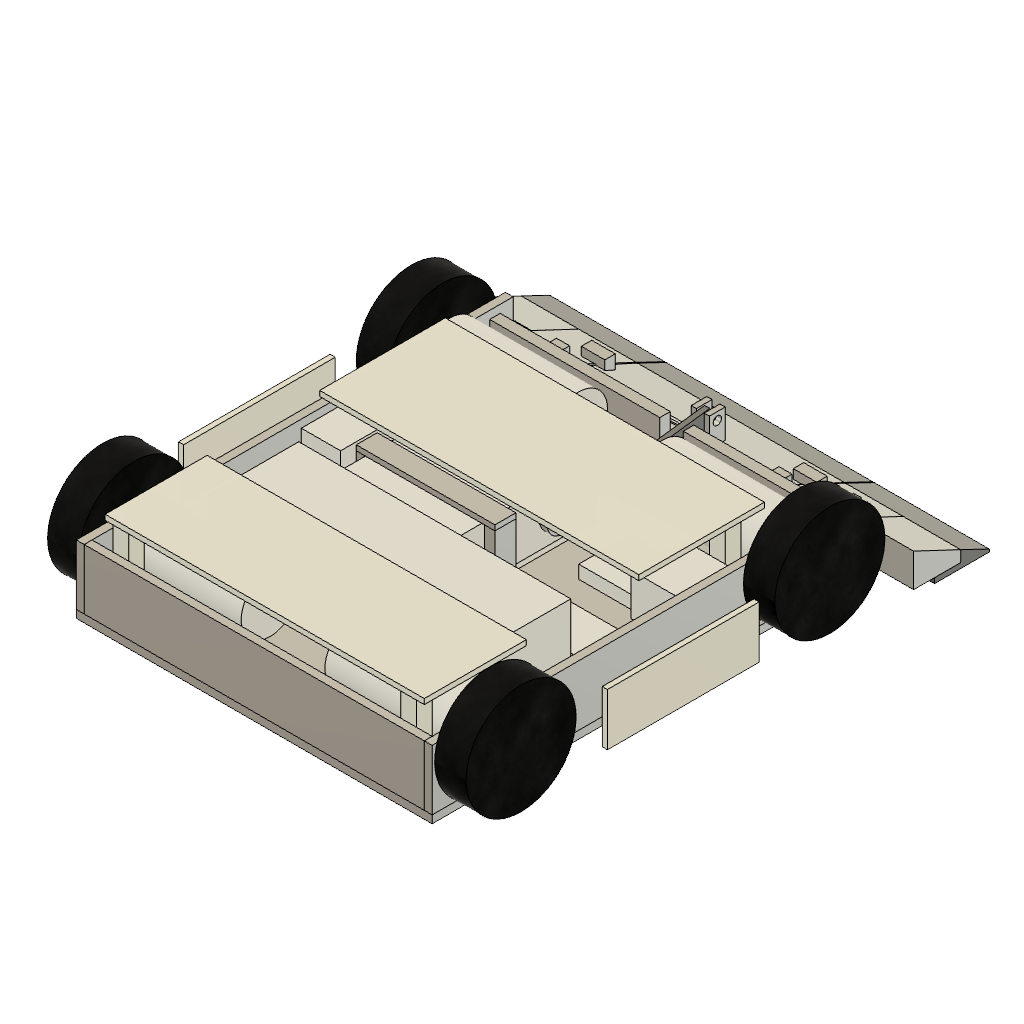
ROBOT_V3_R3_Lifter (Autodesk Fusion 360 design; units mm, degrees)
part number: 2026-09-25-01-00-55-183
part number: 2026-09-25-01-00-55-288
part number: 2026-09-25-01-00-55-293
part number: 2026-09-25-01-00-55-304
part number: 2026-09-25-01-00-55-313
part number: 2026-09-25-01-00-55-323
part number: 2026-09-25-01-00-55-333
part number: 2026-09-25-01-00-55-343
part number: 2026-09-25-01-00-55-353
part number: 2026-09-25-01-00-55-375
part number: 2026-09-25-01-00-55-378
part number: 2026-09-25-01-00-55-389
part number: 2026-09-25-01-00-55-400
part number: 2026-09-25-01-00-55-412
part number: 2026-09-25-01-00-55-424
part number: 2026-09-25-01-00-55-437
part number: 2026-09-25-01-00-55-451
part number: 2026-09-25-01-00-55-467
part number: 2026-09-25-01-00-55-483
part number: 2026-09-25-01-00-55-502
part number: 2026-09-25-01-00-55-522
part number: 2026-09-25-01-00-55-527
part number: 2026-09-25-01-00-55-700
part number: 2026-09-25-01-00-55-756
part number: 2026-09-25-01-00-55-814
part number: 2026-09-25-01-00-55-881
part number: 2026-09-25-01-00-55-947
part number: 2026-09-25-01-00-56-020
part number: 2026-09-25-01-00-56-029
part number: 2026-09-25-01-00-56-371
part number: 2026-09-25-01-00-56-429
part number: 2026-09-25-01-00-56-469
part number: 2026-09-25-01-00-56-511
part number: 2026-09-25-01-00-56-554
part number: 2026-09-25-01-00-56-599
part number: 2026-09-25-01-00-56-645
part number: 2026-09-25-01-00-56-689
part number: 2026-09-25-01-00-56-777
part number: 2026-09-25-01-00-56-983
part number: 2026-09-25-01-00-56-997
part number: 2026-09-25-01-00-57-050
part number: 2026-09-25-01-00-57-102
part number: 2026-09-25-01-00-57-155
part number: 2026-09-25-01-00-57-208
part number: 2026-09-25-01-00-57-261
part number: 2026-09-25-01-00-57-276
part number: 2026-09-25-01-00-57-328
part number: 2026-09-25-01-00-57-386
part number: 2026-09-25-01-00-57-443
part number: 2026-09-25-01-00-57-501
part number: 2026-09-25-01-00-57-558
Autodesk Fusion 360 part; units mm, degrees
sketch "Base_6061_3mm_Footprint" plane through (0, 0, 0) normal (0, 1, 0) x (1, 0, 0) in component "Base_6061_3mm"
  line L0 (-68, -82) -> (68, -82)
  line L1 (68, -82) -> (68, 74)
  line L2 (68, 74) -> (-68, 74)
  line L3 (-68, 74) -> (-68, -82)
extrude "Extrude1" add sketch "Base_6061_3mm_Footprint" along normal blind 3 from surface at 3 makes body 1 in component "Base_6061_3mm"
sketch "Base_Wing_Tab_L_Footprint" plane through (0, 0, 0) normal (0, 1, 0) x (1, 0, 0) in component "Base_Wing_Tab_L"
  line L0 (-68, 74) -> (-41, 74)
  line L1 (-41, 74) -> (-41, 82)
  line L2 (-41, 82) -> (-68, 82)
  line L3 (-68, 82) -> (-68, 74)
extrude "Extrude1'" add sketch "Base_Wing_Tab_L_Footprint" along normal blind 3 from surface at 3 separate body makes body 2 in component "Base_Wing_Tab_L"
sketch "Base_Wing_Tab_R_Footprint" plane through (0, 0, 0) normal (0, 1, 0) x (1, 0, 0) in component "Base_Wing_Tab_R"
  line L0 (41, 74) -> (68, 74)
  line L1 (68, 74) -> (68, 82)
  line L2 (68, 82) -> (41, 82)
  line L3 (41, 82) -> (41, 74)
extrude "Extrude1''" add sketch "Base_Wing_Tab_R_Footprint" along normal blind 3 from surface at 3 separate body makes body 3 in component "Base_Wing_Tab_R"
sketch "Side_Rail_L_6061_Footprint" plane through (0, 0, 0) normal (0, 1, 0) x (1, 0, 0) in component "Side_Rail_L_6061"
  line L0 (-68, -82) -> (-65, -82)
  line L1 (-65, -82) -> (-65, 82)
  line L2 (-65, 82) -> (-68, 82)
  line L3 (-68, 82) -> (-68, -82)
extrude "Extrude1'''" add sketch "Side_Rail_L_6061_Footprint" along normal blind 23 from surface at 6 separate body makes body 4 in component "Side_Rail_L_6061"
sketch "Side_Rail_R_6061_Footprint" plane through (0, 0, 0) normal (0, 1, 0) x (1, 0, 0) in component "Side_Rail_R_6061"
  line L0 (65, -82) -> (68, -82)
  line L1 (68, -82) -> (68, 82)
  line L2 (68, 82) -> (65, 82)
  line L3 (65, 82) -> (65, -82)
extrude "Extrude1''''" add sketch "Side_Rail_R_6061_Footprint" along normal blind 23 from surface at 6 separate body makes body 5 in component "Side_Rail_R_6061"
sketch "Rear_Cross_Member_6061_Footprint" plane through (0, 0, 0) normal (0, 1, 0) x (1, 0, 0) in component "Rear_Cross_Member_6061"
  line L0 (-65, -82) -> (65, -82)
  line L1 (65, -82) -> (65, -79)
  line L2 (65, -79) -> (-65, -79)
  line L3 (-65, -79) -> (-65, -82)
extrude "Extrude1'''''" add sketch "Rear_Cross_Member_6061_Footprint" along normal blind 23 from surface at 6 separate body makes body 6 in component "Rear_Cross_Member_6061"
sketch "Front_Impact_Bulkhead_6061_Footprint" plane through (0, 0, 0) normal (0, 1, 0) x (1, 0, 0) in component "Front_Impact_Bulkhead_6061"
  line L0 (-62, 70) -> (62, 70)
  line L1 (62, 70) -> (62, 74)
  line L2 (62, 74) -> (-62, 74)
  line L3 (-62, 74) -> (-62, 70)
extrude "Extrude1''''''" add sketch "Front_Impact_Bulkhead_6061_Footprint" along normal blind 23 from surface at 6 separate body makes body 7 in component "Front_Impact_Bulkhead_6061"
sketch "Pushrod_Slot" plane through (0, 0, 0) normal (1, 0, 0) x (0, 0, -1) in component "Front_Impact_Bulkhead_6061"
  line L0 (69, 14) -> (69, 30)
  line L1 (69, 30) -> (75, 30)
  line L2 (75, 30) -> (75, 14)
  line L3 (75, 14) -> (69, 14)
extrude "Extrude2" cut sketch "Pushrod_Slot" along normal blind 9 from surface at 3 bodies 7 in component "Front_Impact_Bulkhead_6061"
sketch "BBB_22mm_Gearmotor_ENVELOPE_L_Rear_Section" plane through (0, 0, 0) normal (1, 0, 0) x (0, 0, -1) in component "BBB_22mm_Gearmotor_ENVELOPE_L_Rear"
  circle A0 centre (-60, 23) radius 11
extrude "Extrude1'''''''" add sketch "BBB_22mm_Gearmotor_ENVELOPE_L_Rear_Section" along normal blind 49 from surface at -65 separate body makes body 8 in component "BBB_22mm_Gearmotor_ENVELOPE_L_Rear"
sketch "Wheel_42mm_ENVELOPE_L_Rear_Section" plane through (0, 0, 0) normal (1, 0, 0) x (0, 0, -1) in component "Wheel_42mm_ENVELOPE_L_Rear"
  circle A0 centre (-60, 23) radius 21
extrude "Extrude1''''''''" add sketch "Wheel_42mm_ENVELOPE_L_Rear_Section" along normal blind 12 from surface at -80 separate body makes body 9 in component "Wheel_42mm_ENVELOPE_L_Rear"
sketch "BBB_22mm_Gearmotor_ENVELOPE_L_Front_Section" plane through (0, 0, 0) normal (1, 0, 0) x (0, 0, -1) in component "BBB_22mm_Gearmotor_ENVELOPE_L_Front"
  circle A0 centre (58, 23) radius 11
extrude "Extrude1'''''''''" add sketch "BBB_22mm_Gearmotor_ENVELOPE_L_Front_Section" along normal blind 49 from surface at -65 separate body makes body 10 in component "BBB_22mm_Gearmotor_ENVELOPE_L_Front"
sketch "Wheel_42mm_ENVELOPE_L_Front_Section" plane through (0, 0, 0) normal (1, 0, 0) x (0, 0, -1) in component "Wheel_42mm_ENVELOPE_L_Front"
  circle A0 centre (58, 23) radius 21
extrude "Extrude1''''''''''" add sketch "Wheel_42mm_ENVELOPE_L_Front_Section" along normal blind 12 from surface at -80 separate body makes body 11 in component "Wheel_42mm_ENVELOPE_L_Front"
sketch "BBB_22mm_Gearmotor_ENVELOPE_R_Rear_Section" plane through (0, 0, 0) normal (1, 0, 0) x (0, 0, -1) in component "BBB_22mm_Gearmotor_ENVELOPE_R_Rear"
  circle A0 centre (-60, 23) radius 11
extrude "Extrude1'''''''''''" add sketch "BBB_22mm_Gearmotor_ENVELOPE_R_Rear_Section" along normal blind 49 from surface at 16 separate body makes body 12 in component "BBB_22mm_Gearmotor_ENVELOPE_R_Rear"
sketch "Wheel_42mm_ENVELOPE_R_Rear_Section" plane through (0, 0, 0) normal (1, 0, 0) x (0, 0, -1) in component "Wheel_42mm_ENVELOPE_R_Rear"
  circle A0 centre (-60, 23) radius 21
extrude "Extrude1''''''''''''" add sketch "Wheel_42mm_ENVELOPE_R_Rear_Section" along normal blind 12 from surface at 68 separate body makes body 13 in component "Wheel_42mm_ENVELOPE_R_Rear"
sketch "BBB_22mm_Gearmotor_ENVELOPE_R_Front_Section" plane through (0, 0, 0) normal (1, 0, 0) x (0, 0, -1) in component "BBB_22mm_Gearmotor_ENVELOPE_R_Front"
  circle A0 centre (58, 23) radius 11
extrude "Extrude1'''''''''''''" add sketch "BBB_22mm_Gearmotor_ENVELOPE_R_Front_Section" along normal blind 49 from surface at 16 separate body makes body 14 in component "BBB_22mm_Gearmotor_ENVELOPE_R_Front"
sketch "Wheel_42mm_ENVELOPE_R_Front_Section" plane through (0, 0, 0) normal (1, 0, 0) x (0, 0, -1) in component "Wheel_42mm_ENVELOPE_R_Front"
  circle A0 centre (58, 23) radius 21
extrude "Extrude1''''''''''''''" add sketch "Wheel_42mm_ENVELOPE_R_Front_Section" along normal blind 12 from surface at 68 separate body makes body 15 in component "Wheel_42mm_ENVELOPE_R_Front"
sketch "Replaceable_Side_Guard_L_Footprint" plane through (0, 0, 0) normal (0, 1, 0) x (1, 0, 0) in component "Replaceable_Side_Guard_L"
  line L0 (-82, -29) -> (-80, -29)
  line L1 (-80, -29) -> (-80, 29)
  line L2 (-80, 29) -> (-82, 29)
  line L3 (-82, 29) -> (-82, -29)
extrude "Extrude1'''''''''''''''" add sketch "Replaceable_Side_Guard_L_Footprint" along normal blind 20 from surface at 8 separate body makes body 16 in component "Replaceable_Side_Guard_L"
sketch "Replaceable_Side_Guard_R_Footprint" plane through (0, 0, 0) normal (0, 1, 0) x (1, 0, 0) in component "Replaceable_Side_Guard_R"
  line L0 (80, -29) -> (82, -29)
  line L1 (82, -29) -> (82, 29)
  line L2 (82, 29) -> (80, 29)
  line L3 (80, 29) -> (80, -29)
extrude "Extrude1''''''''''''''''" add sketch "Replaceable_Side_Guard_R_Footprint" along normal blind 20 from surface at 8 separate body makes body 17 in component "Replaceable_Side_Guard_R"
sketch "Wing_Root_Profile" plane through (0, 0, 0) normal (1, 0, 0) x (0, 0, -1) in component "Fixed_Plow_Wings_6061"
  line L0 (74, 6) -> (74, 23)
  line L1 (74, 23) -> (104, 8.79)
  line L2 (104, 8.79) -> (104, 4.5)
  line L3 (104, 4.5) -> (94, 4.5)
  line L4 (94, 4.5) -> (82, 6)
  line L5 (82, 6) -> (74, 6)
extrude "Extrude1'''''''''''''''''" add sketch "Wing_Root_Profile" along normal blind 22 from surface at -62 separate body makes body 18 in component "Fixed_Plow_Wings_6061"
sketch "Wing_Outer_Profile" plane through (0, 0, 0) normal (1, 0, 0) x (0, 0, -1) in component "Fixed_Plow_Wings_6061"
  line L0 (86, 4.5) -> (86, 17.3)
  line L1 (86, 17.3) -> (104, 8.79)
  line L2 (104, 8.79) -> (104, 4.5)
  line L3 (104, 4.5) -> (86, 4.5)
extrude "Extrude2'" add sketch "Wing_Outer_Profile" along normal blind 22 from surface at -84 bodies 18 in component "Fixed_Plow_Wings_6061"
sketch "Up_Stop_Block" plane through (0, 0, 0) normal (1, 0, 0) x (0, 0, -1) in component "Fixed_Plow_Wings_6061"
  line L0 (74, 23) -> (74, 27)
  line L1 (74, 27) -> (78.54, 27)
  line L2 (78.54, 27) -> (78.54, 20.8496)
  line L3 (78.54, 20.8496) -> (74, 23)
extrude "Extrude3" add sketch "Up_Stop_Block" along normal blind 5 from surface at -45 bodies 18 in component "Fixed_Plow_Wings_6061"
sketch "Pivot_Bore_6p4mm" plane through (0, 0, 0) normal (1, 0, 0) x (0, 0, -1) in component "Fixed_Plow_Wings_6061"
  circle A0 centre (80.5, 13) radius 3.2
extrude "Extrude4" cut sketch "Pivot_Bore_6p4mm" along normal blind 6.5 from surface at -46.5 bodies 18 in component "Fixed_Plow_Wings_6061"
sketch "Wing_Root_Profile (1)" plane through (0, 0, 0) normal (1, 0, 0) x (0, 0, -1) in component "Fixed_Plow_Wings_6061"
  line L0 (74, 6) -> (74, 23)
  line L1 (74, 23) -> (104, 8.79)
  line L2 (104, 8.79) -> (104, 4.5)
  line L3 (104, 4.5) -> (94, 4.5)
  line L4 (94, 4.5) -> (82, 6)
  line L5 (82, 6) -> (74, 6)
extrude "Extrude5" add sketch "Wing_Root_Profile (1)" along normal blind 22 from surface at 40 separate body makes body 19 in component "Fixed_Plow_Wings_6061"
sketch "Wing_Outer_Profile (1)" plane through (0, 0, 0) normal (1, 0, 0) x (0, 0, -1) in component "Fixed_Plow_Wings_6061"
  line L0 (86, 4.5) -> (86, 17.3)
  line L1 (86, 17.3) -> (104, 8.79)
  line L2 (104, 8.79) -> (104, 4.5)
  line L3 (104, 4.5) -> (86, 4.5)
extrude "Extrude6" add sketch "Wing_Outer_Profile (1)" along normal blind 22 from surface at 62 bodies 19 in component "Fixed_Plow_Wings_6061"
sketch "Up_Stop_Block (1)" plane through (0, 0, 0) normal (1, 0, 0) x (0, 0, -1) in component "Fixed_Plow_Wings_6061"
  line L0 (74, 23) -> (74, 27)
  line L1 (74, 27) -> (78.54, 27)
  line L2 (78.54, 27) -> (78.54, 20.8496)
  line L3 (78.54, 20.8496) -> (74, 23)
extrude "Extrude7" add sketch "Up_Stop_Block (1)" along normal blind 5 from surface at 40 bodies 19 in component "Fixed_Plow_Wings_6061"
sketch "Pivot_Bore_6p4mm (1)" plane through (0, 0, 0) normal (1, 0, 0) x (0, 0, -1) in component "Fixed_Plow_Wings_6061"
  circle A0 centre (80.5, 13) radius 3.2
extrude "Extrude8" cut sketch "Pivot_Bore_6p4mm (1)" along normal blind 6.5 from surface at 39.5 bodies 19 in component "Fixed_Plow_Wings_6061"
sketch "Wing_Edge_Profile" plane through (0, 0, 0) normal (1, 0, 0) x (0, 0, -1) in component "Wing_Steel_Edges"
  line L0 (94, 2.5) -> (94, 4.5)
  line L1 (94, 4.5) -> (104, 4.5)
  line L2 (104, 4.5) -> (104, 8.79)
  line L3 (104, 8.79) -> (115, 3.5)
  line L4 (115, 3.5) -> (115, 2.5)
  line L5 (115, 2.5) -> (94, 2.5)
extrude "Extrude1''''''''''''''''''" add sketch "Wing_Edge_Profile" along normal blind 44 from surface at -84 separate body makes body 20 in component "Wing_Steel_Edges"
sketch "Wing_Edge_Profile (1)" plane through (0, 0, 0) normal (1, 0, 0) x (0, 0, -1) in component "Wing_Steel_Edges"
  line L0 (94, 2.5) -> (94, 4.5)
  line L1 (94, 4.5) -> (104, 4.5)
  line L2 (104, 4.5) -> (104, 8.79)
  line L3 (104, 8.79) -> (115, 3.5)
  line L4 (115, 3.5) -> (115, 2.5)
  line L5 (115, 2.5) -> (94, 2.5)
extrude "Extrude2''" add sketch "Wing_Edge_Profile (1)" along normal blind 44 from surface at 40 separate body makes body 21 in component "Wing_Steel_Edges"
sketch "M3x20_Bolt_ENVELOPE_x-49.5_Section" plane through (0, 0, 0) normal (0, 0, 1) x (1, 0, 0) in component "M3x20_Bolt_ENVELOPE_x-49.5"
  circle A0 centre (-49.5, 10) radius 1.5
extrude "Extrude1'''''''''''''''''''" add sketch "M3x20_Bolt_ENVELOPE_x-49.5_Section" along normal blind 19 from surface at -86 separate body makes body 22 in component "M3x20_Bolt_ENVELOPE_x-49.5"
sketch "Bolt_Clearance_x-49.5" plane through (0, 0, 0) normal (0, 0, 1) x (1, 0, 0) in component "Front_Impact_Bulkhead_6061"
  circle A0 centre (-49.5, 10) radius 1.7
extrude "Extrude3'" cut sketch "Bolt_Clearance_x-49.5" along normal blind 5 from surface at -74.5 bodies 7 in component "Front_Impact_Bulkhead_6061"
sketch "Bolt_Tapped_x-49.5" plane through (0, 0, 0) normal (0, 0, 1) x (1, 0, 0) in component "Fixed_Plow_Wings_6061"
  circle A0 centre (-49.5, 10) radius 1.5
extrude "Extrude9" cut sketch "Bolt_Tapped_x-49.5" along normal blind 12 from surface at -86 bodies 18 in component "Fixed_Plow_Wings_6061"
sketch "M3x20_Bolt_ENVELOPE_x-58.5_Section" plane through (0, 0, 0) normal (0, 0, 1) x (1, 0, 0) in component "M3x20_Bolt_ENVELOPE_x-58.5"
  circle A0 centre (-58.5, 10) radius 1.5
extrude "Extrude1''''''''''''''''''''" add sketch "M3x20_Bolt_ENVELOPE_x-58.5_Section" along normal blind 19 from surface at -86 separate body makes body 23 in component "M3x20_Bolt_ENVELOPE_x-58.5"
sketch "Bolt_Clearance_x-58.5" plane through (0, 0, 0) normal (0, 0, 1) x (1, 0, 0) in component "Front_Impact_Bulkhead_6061"
  circle A0 centre (-58.5, 10) radius 1.7
extrude "Extrude4'" cut sketch "Bolt_Clearance_x-58.5" along normal blind 5 from surface at -74.5 bodies 7 in component "Front_Impact_Bulkhead_6061"
sketch "Bolt_Tapped_x-58.5" plane through (0, 0, 0) normal (0, 0, 1) x (1, 0, 0) in component "Fixed_Plow_Wings_6061"
  circle A0 centre (-58.5, 10) radius 1.5
extrude "Extrude10" cut sketch "Bolt_Tapped_x-58.5" along normal blind 12 from surface at -86 bodies 18 in component "Fixed_Plow_Wings_6061"
sketch "M3x20_Bolt_ENVELOPE_x+49.5_Section" plane through (0, 0, 0) normal (0, 0, 1) x (1, 0, 0) in component "M3x20_Bolt_ENVELOPE_x+49.5"
  circle A0 centre (49.5, 10) radius 1.5
extrude "Extrude1'''''''''''''''''''''" add sketch "M3x20_Bolt_ENVELOPE_x+49.5_Section" along normal blind 19 from surface at -86 separate body makes body 24 in component "M3x20_Bolt_ENVELOPE_x+49.5"
sketch "Bolt_Clearance_x+49.5" plane through (0, 0, 0) normal (0, 0, 1) x (1, 0, 0) in component "Front_Impact_Bulkhead_6061"
  circle A0 centre (49.5, 10) radius 1.7
extrude "Extrude5'" cut sketch "Bolt_Clearance_x+49.5" along normal blind 5 from surface at -74.5 bodies 7 in component "Front_Impact_Bulkhead_6061"
sketch "Bolt_Tapped_x+49.5" plane through (0, 0, 0) normal (0, 0, 1) x (1, 0, 0) in component "Fixed_Plow_Wings_6061"
  circle A0 centre (49.5, 10) radius 1.5
extrude "Extrude11" cut sketch "Bolt_Tapped_x+49.5" along normal blind 12 from surface at -86 bodies 19 in component "Fixed_Plow_Wings_6061"
sketch "M3x20_Bolt_ENVELOPE_x+58.5_Section" plane through (0, 0, 0) normal (0, 0, 1) x (1, 0, 0) in component "M3x20_Bolt_ENVELOPE_x+58.5"
  circle A0 centre (58.5, 10) radius 1.5
extrude "Extrude1''''''''''''''''''''''" add sketch "M3x20_Bolt_ENVELOPE_x+58.5_Section" along normal blind 19 from surface at -86 separate body makes body 25 in component "M3x20_Bolt_ENVELOPE_x+58.5"
sketch "Bolt_Clearance_x+58.5" plane through (0, 0, 0) normal (0, 0, 1) x (1, 0, 0) in component "Front_Impact_Bulkhead_6061"
  circle A0 centre (58.5, 10) radius 1.7
extrude "Extrude6'" cut sketch "Bolt_Clearance_x+58.5" along normal blind 5 from surface at -74.5 bodies 7 in component "Front_Impact_Bulkhead_6061"
sketch "Bolt_Tapped_x+58.5" plane through (0, 0, 0) normal (0, 0, 1) x (1, 0, 0) in component "Fixed_Plow_Wings_6061"
  circle A0 centre (58.5, 10) radius 1.5
extrude "Extrude12" cut sketch "Bolt_Tapped_x+58.5" along normal blind 12 from surface at -86 bodies 19 in component "Fixed_Plow_Wings_6061"
sketch "Lifter_Profile" plane through (0, 0, 0) normal (1, 0, 0) x (0, 0, -1) in component "Lifting_Wedge_6061"
  line L0 (80.5, 7) -> (80.5, 19.5)
  line L1 (80.5, 19.5) -> (104, 8.79)
  line L2 (104, 8.79) -> (104, 4.5)
  line L3 (104, 4.5) -> (94, 4.5)
  line L4 (94, 4.5) -> (86, 5.5)
  line L5 (86, 5.5) -> (80.5, 7)
extrude "Extrude1'''''''''''''''''''''''" add sketch "Lifter_Profile" along normal blind 79 from surface at -39.5 separate body makes body 26 in component "Lifting_Wedge_6061"
sketch "Pivot_Boss_Section" plane through (0, 0, 0) normal (1, 0, 0) x (0, 0, -1) in component "Lifting_Wedge_6061"
  circle A0 centre (80.5, 13) radius 6
extrude "Extrude2'''" add sketch "Pivot_Boss_Section" along normal blind 79 from surface at -39.5 bodies 26 in component "Lifting_Wedge_6061"
sketch "Pushrod_Clevis" plane through (0, 0, 0) normal (1, 0, 0) x (0, 0, -1) in component "Lifting_Wedge_6061"
  line L0 (81, 17) -> (81, 28)
  line L1 (81, 28) -> (87, 28)
  line L2 (87, 28) -> (87, 17)
  line L3 (87, 17) -> (81, 17)
extrude "Extrude3''" add sketch "Pushrod_Clevis" along normal blind 2 from surface at 4 bodies 26 in component "Lifting_Wedge_6061"
sketch "Pushrod_Clevis (1)" plane through (0, 0, 0) normal (1, 0, 0) x (0, 0, -1) in component "Lifting_Wedge_6061"
  line L0 (81, 17) -> (81, 28)
  line L1 (81, 28) -> (87, 28)
  line L2 (87, 28) -> (87, 17)
  line L3 (87, 17) -> (81, 17)
extrude "Extrude4''" add sketch "Pushrod_Clevis (1)" along normal blind 2 from surface at 9 bodies 26 in component "Lifting_Wedge_6061"
sketch "Down_Stop_Web" plane through (0, 0, 0) normal (1, 0, 0) x (0, 0, -1) in component "Lifting_Wedge_6061"
  line L0 (88, 12) -> (88, 19.6)
  line L1 (88, 19.6) -> (92, 19.6)
  line L2 (92, 19.6) -> (92, 12)
  line L3 (92, 12) -> (88, 12)
extrude "Extrude5''" add sketch "Down_Stop_Web" along normal blind 3.5 from surface at -39.5 bodies 26 in component "Lifting_Wedge_6061"
sketch "Down_Stop_Tab" plane through (0, 0, 0) normal (1, 0, 0) x (0, 0, -1) in component "Lifting_Wedge_6061"
  line L0 (88, 16.3687) -> (88, 19.6)
  line L1 (88, 19.6) -> (92, 19.6)
  line L2 (92, 19.6) -> (92, 14.474)
  line L3 (92, 14.474) -> (88, 16.3687)
extrude "Extrude6''" add sketch "Down_Stop_Tab" along normal blind 5.5 from surface at -45 separate body makes body 27 in component "Lifting_Wedge_6061"
sketch "Down_Stop_Web (1)" plane through (0, 0, 0) normal (1, 0, 0) x (0, 0, -1) in component "Lifting_Wedge_6061"
  line L0 (88, 12) -> (88, 19.6)
  line L1 (88, 19.6) -> (92, 19.6)
  line L2 (92, 19.6) -> (92, 12)
  line L3 (92, 12) -> (88, 12)
extrude "Extrude7'" add sketch "Down_Stop_Web (1)" along normal blind 3.5 from surface at 36 bodies 26 in component "Lifting_Wedge_6061"
sketch "Down_Stop_Tab (1)" plane through (0, 0, 0) normal (1, 0, 0) x (0, 0, -1) in component "Lifting_Wedge_6061"
  line L0 (88, 16.3687) -> (88, 19.6)
  line L1 (88, 19.6) -> (92, 19.6)
  line L2 (92, 19.6) -> (92, 14.474)
  line L3 (92, 14.474) -> (88, 16.3687)
extrude "Extrude8'" add sketch "Down_Stop_Tab (1)" along normal blind 5.5 from surface at 39.5 separate body makes body 28 in component "Lifting_Wedge_6061"
combine "Combine1" operation add target body 26 tool bodies 27 28 in component "Lifting_Wedge_6061"
sketch "Pivot_Bore_6p4mm (2)" plane through (0, 0, 0) normal (1, 0, 0) x (0, 0, -1) in component "Lifting_Wedge_6061"
  circle A0 centre (80.5, 13) radius 3.2
extrude "Extrude9'" cut sketch "Pivot_Bore_6p4mm (2)" along normal mid plane 200 bodies 26 in component "Lifting_Wedge_6061"
sketch "Pushrod_Pin_Bore_3p2mm" plane through (0, 0, 0) normal (1, 0, 0) x (0, 0, -1) in component "Lifting_Wedge_6061"
  circle A0 centre (84, 25) radius 1.6
extrude "Extrude10'" cut sketch "Pushrod_Pin_Bore_3p2mm" along normal mid plane 200 bodies 26 in component "Lifting_Wedge_6061"
sketch "Lifter_Edge_Profile" plane through (0, 0, 0) normal (1, 0, 0) x (0, 0, -1) in component "Lifter_Steel_Edge"
  line L0 (94, 2.5) -> (94, 4.5)
  line L1 (94, 4.5) -> (104, 4.5)
  line L2 (104, 4.5) -> (104, 8.79)
  line L3 (104, 8.79) -> (115, 3.5)
  line L4 (115, 3.5) -> (115, 2.5)
  line L5 (115, 2.5) -> (94, 2.5)
extrude "Extrude1''''''''''''''''''''''''" add sketch "Lifter_Edge_Profile" along normal blind 79 from surface at -39.5 separate body makes body 29 in component "Lifter_Steel_Edge"
sketch "Pivot_Pin_6mm_ENVELOPE_Section" plane through (0, 0, 0) normal (1, 0, 0) x (0, 0, -1) in component "Pivot_Pin_6mm_ENVELOPE"
  circle A0 centre (80.5, 13) radius 3
extrude "Extrude1'''''''''''''''''''''''''" add sketch "Pivot_Pin_6mm_ENVELOPE_Section" along normal blind 92 from surface at -46 separate body makes body 30 in component "Pivot_Pin_6mm_ENVELOPE"
sketch "Repeat_40kg_Servo_56x44p5x20_MAX_Footprint" plane through (0, 0, 0) normal (0, 1, 0) x (1, 0, 0) in component "Repeat_40kg_Servo_56x44p5x20_MAX"
  line L0 (-41.5, -10) -> (3, -10)
  line L1 (3, -10) -> (3, 46.2)
  line L2 (3, 46.2) -> (-41.5, 46.2)
  line L3 (-41.5, 46.2) -> (-41.5, -10)
extrude "Extrude1''''''''''''''''''''''''''" add sketch "Repeat_40kg_Servo_56x44p5x20_MAX_Footprint" along normal blind 20 from surface at 8 separate body makes body 31 in component "Repeat_40kg_Servo_56x44p5x20_MAX"
sketch "Servo_Foam_Pad_2mm_Footprint" plane through (0, 0, 0) normal (0, 1, 0) x (1, 0, 0) in component "Servo_Foam_Pad_2mm"
  line L0 (-41.5, -10) -> (3, -10)
  line L1 (3, -10) -> (3, 46.2)
  line L2 (3, 46.2) -> (-41.5, 46.2)
  line L3 (-41.5, 46.2) -> (-41.5, -10)
extrude "Extrude1'''''''''''''''''''''''''''" add sketch "Servo_Foam_Pad_2mm_Footprint" along normal blind 2 from surface at 6 separate body makes body 32 in component "Servo_Foam_Pad_2mm"
sketch "Servo_Hold_Down_Strap_6061_Footprint" plane through (0, 0, 0) normal (0, 1, 0) x (1, 0, 0) in component "Servo_Hold_Down_Strap_6061"
  line L0 (-45, 2) -> (8, 2)
  line L1 (8, 2) -> (8, 10)
  line L2 (8, 10) -> (-45, 10)
  line L3 (-45, 10) -> (-45, 2)
extrude "Extrude1''''''''''''''''''''''''''''" add sketch "Servo_Hold_Down_Strap_6061_Footprint" along normal blind 2 from surface at 28 separate body makes body 33 in component "Servo_Hold_Down_Strap_6061"
sketch "Servo_Strap_Post_L_6061_Footprint" plane through (0, 0, 0) normal (0, 1, 0) x (1, 0, 0) in component "Servo_Strap_Post_L_6061"
  line L0 (-45, 2) -> (-42, 2)
  line L1 (-42, 2) -> (-42, 10)
  line L2 (-42, 10) -> (-45, 10)
  line L3 (-45, 10) -> (-45, 2)
extrude "Extrude1'''''''''''''''''''''''''''''" add sketch "Servo_Strap_Post_L_6061_Footprint" along normal blind 22 from surface at 6 separate body makes body 34 in component "Servo_Strap_Post_L_6061"
sketch "Servo_Strap_Post_R_6061_Footprint" plane through (0, 0, 0) normal (0, 1, 0) x (1, 0, 0) in component "Servo_Strap_Post_R_6061"
  line L0 (4, 2) -> (8, 2)
  line L1 (8, 2) -> (8, 10)
  line L2 (8, 10) -> (4, 10)
  line L3 (4, 10) -> (4, 2)
extrude "Extrude1''''''''''''''''''''''''''''''" add sketch "Servo_Strap_Post_R_6061_Footprint" along normal blind 22 from surface at 6 separate body makes body 35 in component "Servo_Strap_Post_R_6061"
sketch "Sketch1" plane through (0, 0, 0) normal (1, 0, 0) x (0, 0, -1) in component "Servo_Crank_Arm_6061"
  line L0 (29.5501, 21.471) -> (41.4505, 23.0136)
  line L1 (41.4505, 23.0136) -> (42.3504, 16.0717)
  line L2 (42.3504, 16.0717) -> (30.4499, 14.529)
  line L3 (30.4499, 14.529) -> (29.5501, 21.471)
extrude "Extrude1'''''''''''''''''''''''''''''''" add sketch "Sketch1" along normal blind 3 from surface at 3 separate body makes body 36 in component "Servo_Crank_Arm_6061"
sketch "Crank_Hub_Section" plane through (0, 0, 0) normal (1, 0, 0) x (0, 0, -1) in component "Servo_Crank_Arm_6061"
  circle A0 centre (30, 18) radius 6
extrude "Extrude2''''" add sketch "Crank_Hub_Section" along normal blind 3 from surface at 3 bodies 36 in component "Servo_Crank_Arm_6061"
sketch "Sketch1 (2)" plane through (0, 0, 0) normal (1, 0, 0) x (0, 0, -1) in component "Pushrod_Steel_2mm"
  line L0 (41.5148, 22.5178) -> (83.6143, 27.9751)
  line L1 (83.6143, 27.9751) -> (84.3857, 22.0249)
  line L2 (84.3857, 22.0249) -> (42.2861, 16.5675)
  line L3 (42.2861, 16.5675) -> (41.5148, 22.5178)
extrude "Extrude1''''''''''''''''''''''''''''''''" add sketch "Sketch1 (2)" along normal blind 2 from surface at 6.5 separate body makes body 37 in component "Pushrod_Steel_2mm"
sketch "3S_Battery_104x35x27_ENVELOPE_Footprint" plane through (0, 0, 0) normal (0, 1, 0) x (1, 0, 0) in component "3S_Battery_104x35x27_ENVELOPE"
  line L0 (-52, -48) -> (52, -48)
  line L1 (52, -48) -> (52, -13)
  line L2 (52, -13) -> (-52, -13)
  line L3 (-52, -13) -> (-52, -48)
extrude "Extrude1'''''''''''''''''''''''''''''''''" add sketch "3S_Battery_104x35x27_ENVELOPE_Footprint" along normal blind 27 from surface at 8 separate body makes body 38 in component "3S_Battery_104x35x27_ENVELOPE"
sketch "RadioMaster_ER6_Receiver_43x25x15_Footprint" plane through (0, 0, 0) normal (0, 1, 0) x (1, 0, 0) in component "RadioMaster_ER6_Receiver_43x25x15"
  line L0 (-60, -4) -> (-45, -4)
  line L1 (-45, -4) -> (-45, 39)
  line L2 (-45, 39) -> (-60, 39)
  line L3 (-60, 39) -> (-60, -4)
extrude "Extrude1''''''''''''''''''''''''''''''''''" add sketch "RadioMaster_ER6_Receiver_43x25x15_Footprint" along normal blind 25 from surface at 6 separate body makes body 39 in component "RadioMaster_ER6_Receiver_43x25x15"
sketch "BBB_Dual_ESC_v2_ENVELOPE_Footprint" plane through (0, 0, 0) normal (0, 1, 0) x (1, 0, 0) in component "BBB_Dual_ESC_v2_ENVELOPE"
  line L0 (18, 24) -> (42, 24)
  line L1 (42, 24) -> (42, 44)
  line L2 (42, 44) -> (18, 44)
  line L3 (18, 44) -> (18, 24)
extrude "Extrude1'''''''''''''''''''''''''''''''''''" add sketch "BBB_Dual_ESC_v2_ENVELOPE_Footprint" along normal blind 5 from surface at 6 separate body makes body 40 in component "BBB_Dual_ESC_v2_ENVELOPE"
sketch "Hobbywing_UBEC_5A_50x17x10_Footprint" plane through (0, 0, 0) normal (0, 1, 0) x (1, 0, 0) in component "Hobbywing_UBEC_5A_50x17x10"
  line L0 (12, -12) -> (62, -12)
  line L1 (62, -12) -> (62, 5)
  line L2 (62, 5) -> (12, 5)
  line L3 (12, 5) -> (12, -12)
extrude "Extrude1''''''''''''''''''''''''''''''''''''" add sketch "Hobbywing_UBEC_5A_50x17x10_Footprint" along normal blind 10 from surface at 6 separate body makes body 41 in component "Hobbywing_UBEC_5A_50x17x10"
sketch "Power_Switch_ENVELOPE_Footprint" plane through (0, 0, 0) normal (0, 1, 0) x (1, 0, 0) in component "Power_Switch_ENVELOPE"
  line L0 (44, 18) -> (62, 18)
  line L1 (62, 18) -> (62, 38)
  line L2 (62, 38) -> (44, 38)
  line L3 (44, 38) -> (44, 18)
extrude "Extrude1'''''''''''''''''''''''''''''''''''''" add sketch "Power_Switch_ENVELOPE_Footprint" along normal blind 16 from surface at 9 separate body makes body 42 in component "Power_Switch_ENVELOPE"
sketch "Cover_Standoff_L_Rear_Footprint" plane through (0, 0, 0) normal (0, 1, 0) x (1, 0, 0) in component "Cover_Standoff_L_Rear"
  line L0 (-58, -78) -> (-52, -78)
  line L1 (-52, -78) -> (-52, -72)
  line L2 (-52, -72) -> (-58, -72)
  line L3 (-58, -72) -> (-58, -78)
extrude "Extrude1''''''''''''''''''''''''''''''''''''''" add sketch "Cover_Standoff_L_Rear_Footprint" along normal blind 31 from surface at 6 separate body makes body 43 in component "Cover_Standoff_L_Rear"
sketch "Cover_Standoff_L_Front_Footprint" plane through (0, 0, 0) normal (0, 1, 0) x (1, 0, 0) in component "Cover_Standoff_L_Front"
  line L0 (-58, 40) -> (-52, 40)
  line L1 (-52, 40) -> (-52, 46)
  line L2 (-52, 46) -> (-58, 46)
  line L3 (-58, 46) -> (-58, 40)
extrude "Extrude1'''''''''''''''''''''''''''''''''''''''" add sketch "Cover_Standoff_L_Front_Footprint" along normal blind 31 from surface at 6 separate body makes body 44 in component "Cover_Standoff_L_Front"
sketch "Cover_Standoff_R_Rear_Footprint" plane through (0, 0, 0) normal (0, 1, 0) x (1, 0, 0) in component "Cover_Standoff_R_Rear"
  line L0 (52, -78) -> (58, -78)
  line L1 (58, -78) -> (58, -72)
  line L2 (58, -72) -> (52, -72)
  line L3 (52, -72) -> (52, -78)
extrude "Extrude1''''''''''''''''''''''''''''''''''''''''" add sketch "Cover_Standoff_R_Rear_Footprint" along normal blind 31 from surface at 6 separate body makes body 45 in component "Cover_Standoff_R_Rear"
sketch "Cover_Standoff_R_Front_Footprint" plane through (0, 0, 0) normal (0, 1, 0) x (1, 0, 0) in component "Cover_Standoff_R_Front"
  line L0 (52, 40) -> (58, 40)
  line L1 (58, 40) -> (58, 46)
  line L2 (58, 46) -> (52, 46)
  line L3 (52, 46) -> (52, 40)
extrude "Extrude1'''''''''''''''''''''''''''''''''''''''''" add sketch "Cover_Standoff_R_Front_Footprint" along normal blind 31 from surface at 6 separate body makes body 46 in component "Cover_Standoff_R_Front"
sketch "Rear_Service_Lid_2mm_Footprint" plane through (0, 0, 0) normal (0, 1, 0) x (1, 0, 0) in component "Rear_Service_Lid_2mm"
  line L0 (-61, -78) -> (61, -78)
  line L1 (61, -78) -> (61, -39)
  line L2 (61, -39) -> (-61, -39)
  line L3 (-61, -39) -> (-61, -78)
extrude "Extrude1''''''''''''''''''''''''''''''''''''''''''" add sketch "Rear_Service_Lid_2mm_Footprint" along normal blind 2 from surface at 37 separate body makes body 47 in component "Rear_Service_Lid_2mm"
sketch "Center_Service_Lid_2mm_Footprint" plane through (0, 0, 0) normal (0, 1, 0) x (1, 0, 0) in component "Center_Service_Lid_2mm"
  line L0 (-61, 4) -> (61, 4)
  line L1 (61, 4) -> (61, 52)
  line L2 (61, 52) -> (-61, 52)
  line L3 (-61, 52) -> (-61, 4)
extrude "Extrude1'''''''''''''''''''''''''''''''''''''''''''" add sketch "Center_Service_Lid_2mm_Footprint" along normal blind 2 from surface at 37 separate body makes body 48 in component "Center_Service_Lid_2mm"
component "01_Low_Tub_Chassis" placed x (1, 0, 0) y (0, 1, 0) z (0, 0, 1) at (0, 0, 0)
component "02_Four_Wheel_Drive" placed x (1, 0, 0) y (0, 1, 0) z (0, 0, 1) at (0, 0, 0)
component "03_Front_Fixed_Wings" placed x (1, 0, 0) y (0, 1, 0) z (0, 0, 1) at (0, 0, 0)
component "04_Servo_Lifting_Wedge" placed x (1, 0, 0) y (0, 1, 0) z (0, 0, 1) at (0, 0, 0)
component "05_Protected_Electronics_ENVELOPES" placed x (1, 0, 0) y (0, 1, 0) z (0, 0, 1) at (0, 0, 0)
component "06_Removable_Covers" placed x (1, 0, 0) y (0, 1, 0) z (0, 0, 1) at (0, 0, 0)
component "Base_6061_3mm" placed x (1, 0, 0) y (0, 1, 0) z (0, 0, 1) at (0, 0, 0) in component "01_Low_Tub_Chassis"
component "Base_Wing_Tab_L" placed x (1, 0, 0) y (0, 1, 0) z (0, 0, 1) at (0, 0, 0) in component "01_Low_Tub_Chassis"
component "Base_Wing_Tab_R" placed x (1, 0, 0) y (0, 1, 0) z (0, 0, 1) at (0, 0, 0) in component "01_Low_Tub_Chassis"
component "Side_Rail_L_6061" placed x (1, 0, 0) y (0, 1, 0) z (0, 0, 1) at (0, 0, 0) in component "01_Low_Tub_Chassis"
component "Side_Rail_R_6061" placed x (1, 0, 0) y (0, 1, 0) z (0, 0, 1) at (0, 0, 0) in component "01_Low_Tub_Chassis"
component "Rear_Cross_Member_6061" placed x (1, 0, 0) y (0, 1, 0) z (0, 0, 1) at (0, 0, 0) in component "01_Low_Tub_Chassis"
component "Front_Impact_Bulkhead_6061" placed x (1, 0, 0) y (0, 1, 0) z (0, 0, 1) at (0, 0, 0) in component "01_Low_Tub_Chassis"
component "BBB_22mm_Gearmotor_ENVELOPE_L_Rear" placed x (1, 0, 0) y (0, 1, 0) z (0, 0, 1) at (0, 0, 0) in component "02_Four_Wheel_Drive"
component "Wheel_42mm_ENVELOPE_L_Rear" placed x (1, 0, 0) y (0, 1, 0) z (0, 0, 1) at (0, 0, 0) in component "02_Four_Wheel_Drive"
component "BBB_22mm_Gearmotor_ENVELOPE_L_Front" placed x (1, 0, 0) y (0, 1, 0) z (0, 0, 1) at (0, 0, 0) in component "02_Four_Wheel_Drive"
component "Wheel_42mm_ENVELOPE_L_Front" placed x (1, 0, 0) y (0, 1, 0) z (0, 0, 1) at (0, 0, 0) in component "02_Four_Wheel_Drive"
component "BBB_22mm_Gearmotor_ENVELOPE_R_Rear" placed x (1, 0, 0) y (0, 1, 0) z (0, 0, 1) at (0, 0, 0) in component "02_Four_Wheel_Drive"
component "Wheel_42mm_ENVELOPE_R_Rear" placed x (1, 0, 0) y (0, 1, 0) z (0, 0, 1) at (0, 0, 0) in component "02_Four_Wheel_Drive"
component "BBB_22mm_Gearmotor_ENVELOPE_R_Front" placed x (1, 0, 0) y (0, 1, 0) z (0, 0, 1) at (0, 0, 0) in component "02_Four_Wheel_Drive"
component "Wheel_42mm_ENVELOPE_R_Front" placed x (1, 0, 0) y (0, 1, 0) z (0, 0, 1) at (0, 0, 0) in component "02_Four_Wheel_Drive"
component "Replaceable_Side_Guard_L" placed x (1, 0, 0) y (0, 1, 0) z (0, 0, 1) at (0, 0, 0) in component "02_Four_Wheel_Drive"
component "Replaceable_Side_Guard_R" placed x (1, 0, 0) y (0, 1, 0) z (0, 0, 1) at (0, 0, 0) in component "02_Four_Wheel_Drive"
component "Fixed_Plow_Wings_6061" placed x (1, 0, 0) y (0, 1, 0) z (0, 0, 1) at (0, 0, 0) in component "03_Front_Fixed_Wings"
component "Wing_Steel_Edges" placed x (1, 0, 0) y (0, 1, 0) z (0, 0, 1) at (0, 0, 0) in component "03_Front_Fixed_Wings"
component "M3x20_Bolt_ENVELOPE_x-49.5" placed x (1, 0, 0) y (0, 1, 0) z (0, 0, 1) at (0, 0, 0) in component "03_Front_Fixed_Wings"
component "M3x20_Bolt_ENVELOPE_x-58.5" placed x (1, 0, 0) y (0, 1, 0) z (0, 0, 1) at (0, 0, 0) in component "03_Front_Fixed_Wings"
component "M3x20_Bolt_ENVELOPE_x+49.5" placed x (1, 0, 0) y (0, 1, 0) z (0, 0, 1) at (0, 0, 0) in component "03_Front_Fixed_Wings"
component "M3x20_Bolt_ENVELOPE_x+58.5" placed x (1, 0, 0) y (0, 1, 0) z (0, 0, 1) at (0, 0, 0) in component "03_Front_Fixed_Wings"
component "Lifting_Wedge_6061" placed x (1, 0, 0) y (0, 1, 0) z (0, 0, 1) at (0, 0, 0) in component "04_Servo_Lifting_Wedge"
component "Lifter_Steel_Edge" placed x (1, 0, 0) y (0, 1, 0) z (0, 0, 1) at (0, 0, 0) in component "04_Servo_Lifting_Wedge"
component "Pivot_Pin_6mm_ENVELOPE" placed x (1, 0, 0) y (0, 1, 0) z (0, 0, 1) at (0, 0, 0) in component "04_Servo_Lifting_Wedge"
component "Repeat_40kg_Servo_56x44p5x20_MAX" placed x (1, 0, 0) y (0, 1, 0) z (0, 0, 1) at (0, 0, 0) in component "04_Servo_Lifting_Wedge"
component "Servo_Foam_Pad_2mm" placed x (1, 0, 0) y (0, 1, 0) z (0, 0, 1) at (0, 0, 0) in component "04_Servo_Lifting_Wedge"
component "Servo_Hold_Down_Strap_6061" placed x (1, 0, 0) y (0, 1, 0) z (0, 0, 1) at (0, 0, 0) in component "04_Servo_Lifting_Wedge"
component "Servo_Strap_Post_L_6061" placed x (1, 0, 0) y (0, 1, 0) z (0, 0, 1) at (0, 0, 0) in component "04_Servo_Lifting_Wedge"
component "Servo_Strap_Post_R_6061" placed x (1, 0, 0) y (0, 1, 0) z (0, 0, 1) at (0, 0, 0) in component "04_Servo_Lifting_Wedge"
component "Servo_Crank_Arm_6061" placed x (1, 0, 0) y (0, 1, 0) z (0, 0, 1) at (0, 0, 0) in component "04_Servo_Lifting_Wedge"
component "Pushrod_Steel_2mm" placed x (1, 0, 0) y (0, 1, 0) z (0, 0, 1) at (0, 0, 0) in component "04_Servo_Lifting_Wedge"
component "3S_Battery_104x35x27_ENVELOPE" placed x (1, 0, 0) y (0, 1, 0) z (0, 0, 1) at (0, 0, 0) in component "05_Protected_Electronics_ENVELOPES"
component "RadioMaster_ER6_Receiver_43x25x15" placed x (1, 0, 0) y (0, 1, 0) z (0, 0, 1) at (0, 0, 0) in component "05_Protected_Electronics_ENVELOPES"
component "BBB_Dual_ESC_v2_ENVELOPE" placed x (1, 0, 0) y (0, 1, 0) z (0, 0, 1) at (0, 0, 0) in component "05_Protected_Electronics_ENVELOPES"
component "Hobbywing_UBEC_5A_50x17x10" placed x (1, 0, 0) y (0, 1, 0) z (0, 0, 1) at (0, 0, 0) in component "05_Protected_Electronics_ENVELOPES"
component "Power_Switch_ENVELOPE" placed x (1, 0, 0) y (0, 1, 0) z (0, 0, 1) at (0, 0, 0) in component "05_Protected_Electronics_ENVELOPES"
component "Cover_Standoff_L_Rear" placed x (1, 0, 0) y (0, 1, 0) z (0, 0, 1) at (0, 0, 0) in component "06_Removable_Covers"
component "Cover_Standoff_L_Front" placed x (1, 0, 0) y (0, 1, 0) z (0, 0, 1) at (0, 0, 0) in component "06_Removable_Covers"
component "Cover_Standoff_R_Rear" placed x (1, 0, 0) y (0, 1, 0) z (0, 0, 1) at (0, 0, 0) in component "06_Removable_Covers"
component "Cover_Standoff_R_Front" placed x (1, 0, 0) y (0, 1, 0) z (0, 0, 1) at (0, 0, 0) in component "06_Removable_Covers"
component "Rear_Service_Lid_2mm" placed x (1, 0, 0) y (0, 1, 0) z (0, 0, 1) at (0, 0, 0) in component "06_Removable_Covers"
component "Center_Service_Lid_2mm" placed x (1, 0, 0) y (0, 1, 0) z (0, 0, 1) at (0, 0, 0) in component "06_Removable_Covers"
named bodies: "Base_6061_3mm", "Base_Wing_Tab_L", "Base_Wing_Tab_R", "Side_Rail_L_6061", "Side_Rail_R_6061", "Rear_Cross_Member_6061", "Front_Impact_Bulkhead_6061", "BBB_22mm_Gearmotor_ENVELOPE_L_Rear", "Wheel_42mm_ENVELOPE_L_Rear", "BBB_22mm_Gearmotor_ENVELOPE_L_Front", "Wheel_42mm_ENVELOPE_L_Front", "BBB_22mm_Gearmotor_ENVELOPE_R_Rear", "Wheel_42mm_ENVELOPE_R_Rear", "BBB_22mm_Gearmotor_ENVELOPE_R_Front", "Wheel_42mm_ENVELOPE_R_Front", "Replaceable_Side_Guard_L", "Replaceable_Side_Guard_R", "Plow_Wing_L", "Plow_Wing_R", "Wing_Steel_Edge_L", "Wing_Steel_Edge_R", "M3x20_Bolt_ENVELOPE_x-49.5", "M3x20_Bolt_ENVELOPE_x-58.5", "M3x20_Bolt_ENVELOPE_x+49.5", "M3x20_Bolt_ENVELOPE_x+58.5", "Lifting_Wedge_79mm", "Lifter_Steel_Edge_1mm_Tip", "Pivot_Pin_6mm_ENVELOPE", "Repeat_40kg_Servo_56x44p5x20_MAX", "Servo_Foam_Pad_2mm", "Servo_Hold_Down_Strap_6061", "Servo_Strap_Post_L_6061", "Servo_Strap_Post_R_6061", "Servo_Crank_Arm_6061", "Pushrod_Steel_2mm", "3S_Battery_104x35x27_ENVELOPE", "RadioMaster_ER6_Receiver_43x25x15", "BBB_Dual_ESC_v2_ENVELOPE", "Hobbywing_UBEC_5A_50x17x10", "Power_Switch_ENVELOPE", "Cover_Standoff_L_Rear", "Cover_Standoff_L_Front", "Cover_Standoff_R_Rear", "Cover_Standoff_R_Front", "Rear_Service_Lid_2mm", "Center_Service_Lid_2mm"
